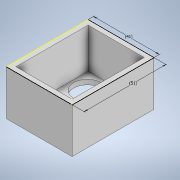
# Autodesk Inventor part: ultrasonido
Saved by Autodesk Inventor 2021 (Build 250183000, 183)
## iProperties
Created: 2024-01-19
Part Number: ultrasonido
Material: Generic
Document SubType Name: Modeling
Designer: MARCO BRAVO
Density: 1 g/cm^3
Appearance: Default
Author: MARCO BRAVO
Autodesk Inventor part; units mm, degrees
ref_plane "YZ Plane" through (0, 0, 0) normal (1, 0, 0) x (0, 1, 0)
ref_plane "XZ Plane" through (0, 0, 0) normal (0, 1, 0) x (-1, 0, 0)
ref_plane "XY Plane" through (0, 0, 0) normal (0, 0, 1) x (1, 0, 0)
sketch "Sketch3" plane through (0, 0, 0) normal (0, 1, 0) x (-1, 0, 0)
  line L0 (0, 0) -> (35, 0)
  line L1 (35, 0) -> (35, -45)
  line L2 (35, -45) -> (0, -45)
  line L3 (0, -45) -> (0, 0)
  circle A0 centre (25, -10.5) radius 8.5
  circle A1 centre (25, -34.5) radius 8.5
  line L4 (35, 0) -> (38, 0)
  line L5 (38, 0) -> (38, -45)
  line L6 (38, -45) -> (38, -48)
  line L7 (38, -48) -> (0, -48)
  line L8 (0, -48) -> (-3, -48)
  line L9 (-3, -48) -> (-3, 0)
  line L10 (-3, 0) -> (-3, 3)
  line L11 (-3, 3) -> (38, 3)
  line L12 (38, 3) -> (38, 0)
  dimension "d26" = 45
  dimension "d27" = 35
  dimension "d31" = 17
  dimension "d32" = 17
  dimension "d33" = 3
  dimension "d34" = 3
  dimension "d35" = 3
  dimension "d36" = 3
  constraints: 26 end point, 5 point on line, 4 perpendicular, 3 parallel, 2 centre point, 2 horizontal, 1 collinear
  measures "d26" distance of L0.end L1.end
  measures "d27" distance of L1.end L2.end
  measures "d31" diameter of A0
  measures "d32" diameter of A1
  measures "d33" distance of L0.end L4.end
  measures "d34" distance of L5.end L6.end
  measures "d35" distance of L7.end L8.end
  measures "d36" distance of L9.end L10.end
extrude "Extrusion3" add sketch "Sketch3" along normal blind 3 contours L0 L1 L2 L3
extrude "Extrusion4" add sketch "Sketch3" along normal blind 28 contours L5 L6 L7 L8 L9 L10 L11 L12
sketch "Sketch4" plane through (0, 28, 0) normal (0, 1, 0) x (1, 0, 0)
  line L0 (-38, 48) -> (-38, -3) projected
  line L1 (-38, -3) -> (2.7105, -3)
  line L2 (-38, -3) -> (3, -3) projected
  line L3 (3, 48) -> (-38, 48) projected
  line L4 (3, -3) -> (3, 48)
  line L5 (-38, 48) -> (3, 48)
  point P0 (0, 0)
  dimension "d41" = 51
  dimension "d43" = 41
  constraints: 6 end point, 2 horizontal, 1 vertical
  measures "d41" distance of L2.end L3.start
  measures "d43" distance of L3.start L0.start
body "Solid2"
